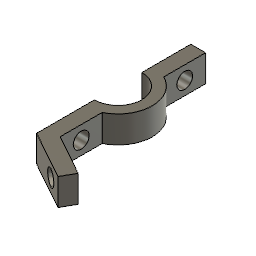
Trumpet+Clamp+1+Secondary (Autodesk Fusion 360 design; units mm, degrees)
Autodesk Fusion 360 part; units mm, degrees
sketch "Sketch1" plane through (0, 0, 0) normal (0, 1, 0) x (1, 0, 0)
  circle A0 centre (0, 0) radius 6.755
  circle A1 centre (0, 0) radius 9.755
  line L0 (0, 0) -> (-9.755, 0) construction
  line L1 (0, 0) -> (9.755, 0) construction
  line L2 (-4.25, -25.7687) -> (18.9274, -38.7154)
  line L3 (4.25, -20.7805) -> (23.0726, -31.2946)
  circle A2 centre (21, -35.005) radius 4.25
  line L4 (21, -35.005) -> (18.9274, -38.7154) construction
  line L5 (21, -35.005) -> (23.0726, -31.2946) construction
  circle A3 centre (21, -35.005) radius 2.25
  line L6 (-4.25, -25.7687) -> (-4.25, -8.7805)
  line L7 (4.25, -20.7805) -> (4.25, -8.7805)
  line L8 (0, 0) -> (0, -20.7805) construction
  line L9 (4.25, -20.7805) -> (-4.25, -20.7805) construction
  line L10 (-4.25, 8.7805) -> (-4.25, 20.7805)
  line L11 (-4.25, 20.7805) -> (4.25, 20.7805)
  line L12 (4.25, 20.7805) -> (4.25, 8.7805)
  line L13 (-4.25, -8.7805) -> (-4.25, 8.7805) construction
  line L14 (4.25, 8.7805) -> (4.25, -8.7805) construction
  line L15 (21, -35.005) -> (21, -39.255) construction
  point P0 (0, -9.755)
  point P1 (21, -39.255)
  dimension "d1" = 13.51
  dimension "d3" = 4.5
  dimension "d4" = 8.5
  dimension "d5" = 21
  dimension "d19" = 8.5
  dimension "d22" = 19.51
  dimension "d31" = 12
  dimension "d32" = 12
  dimension "d35" = 29.5
  constraint coincident A0.centre A1.centre
  constraint concentric A0 A1
  constraint coincident A1 L0.end
  constraint horizontal L0
  constraint coincident A1 L1.end
  constraint parallel L0 L1
  constraint coincident A2.centre L4.start
  constraint coincident A2 L2.end
  constraint coincident A2 L3.end
  constraint parallel L4 L5
  constraint coincident L2.end L4.end
  constraint coincident L3.end L5.end
  constraint coincident A1 L6.end
  constraint coincident A1 L7.end
  constraint parallel L2 L3
  constraint vertical L6
  constraint vertical L7
  constraint vertical L8
  constraint tangent L3 A2
  constraint coincident L6 L9.end
  constraint perpendicular L6 L9
  constraint midpoint L8.end L9
  constraint coincident A1 L10.start
  constraint vertical L10
  constraint perpendicular L10 L11
  constraint coincident A1 L12.end
  constraint perpendicular L11 L12
  constraint vertical L13
  constraint vertical L14
  constraint coincident L8 P0
  constraint coincident A1 P0
  constraint coincident A2 P1
  constraint vertical L15
  constraint coincident P1 L15.end
  measures "d1" diameter of A0
  measures "d3" diameter of A3
  measures "d4" diameter of A2
  measures "d5" horizontal distance of A0.centre A2.centre
  measures "d19" distance of L6 L7
  measures "d22" diameter of A1
  measures "d31" distance of L11.end L12.end
  measures "d32" distance of L3.start L7.end
  measures "d35" vertical distance of P0 P1
extrude "Extrude1" add sketch "Sketch1" along normal blind 7.7
sketch "Sketch2" plane through (-7.8365, 0, 14.0291) normal (0.487666, 0, -0.87303) x (-0.87303, 0, -0.487666)
  line L0 (-35.4044, 0) -> (-13.8443, 0)
  line L1 (-13.8443, 0) -> (-13.8443, 7.7)
  line L2 (-13.8443, 7.7) -> (-35.4044, 7.7)
  line L3 (-35.4044, 7.7) -> (-35.4044, 0)
  line L4 (-13.8443, 3.85) -> (-35.4044, 3.85) construction
  circle A0 centre (-21.8443, 3.85) radius 2.25
  dimension "d33" = 8
  dimension "d34" = 4.5
  constraint midpoint L1 L4.start
  constraint midpoint L3 L4.end
  constraint coincident L4 A0.centre
  measures "d33" distance of L1 A0.centre
  measures "d34" diameter of A0
extrude "Extrude2" cut sketch "Sketch2" against normal up to surface (8.5 mm away) contours A0
sketch "Sketch3" plane through (4.25, 0, 0) normal (1, 0, 0) x (0, 0, -1)
  line L0 (-20.7805, 0) -> (-8.7805, 0)
  line L1 (-8.7805, 0) -> (-8.7805, 7.7)
  line L2 (-8.7805, 7.7) -> (-20.7805, 7.7)
  line L3 (-20.7805, 7.7) -> (-20.7805, 0)
  line L4 (-8.7805, 3.85) -> (-20.7805, 3.85) construction
  circle A0 centre (-14.7805, 3.85) radius 2.25
  line L5 (8.7805, 0) -> (20.7805, 0) construction
  line L6 (20.7805, 0) -> (20.7805, 7.7) construction
  line L7 (20.7805, 7.7) -> (8.7805, 7.7) construction
  line L8 (8.7805, 7.7) -> (8.7805, 0) construction
  line L9 (8.7805, 3.85) -> (20.7805, 3.85) construction
  circle A1 centre (14.7805, 3.85) radius 2.25
  dimension "d16" = 4.5
  constraint midpoint L1 L4.start
  constraint midpoint L3 L4.end
  constraint midpoint L4 A0.centre
  constraint midpoint L8 L9.start
  constraint midpoint L6 L9.end
  constraint midpoint L9 A1.centre
  constraint equal A0 A1
  measures "d16" diameter of A0
extrude "Extrude3" cut sketch "Sketch3" against normal up to surface (8.5 mm away) contours A0 | A1
sketch "Sketch4" plane through (0, 0, 0) normal (1, 0, 0) x (0, 0, -1)
  circle A0 centre (-14.7805, 3.85) radius 2.25 construction
  line L0 (-20.7805, 0) -> (-8.7805, 0) construction
  line L1 (-8.7805, 0) -> (-8.7805, 7.7) construction
  line L2 (-8.7805, 7.7) -> (-20.7805, 7.7) construction
  line L3 (-20.7805, 7.7) -> (-20.7805, 0) construction
  line L4 (8.7805, 0) -> (-8.7805, 0) construction
  line L5 (-8.7805, 0) -> (-8.7805, 7.7) construction
  line L6 (8.7805, 7.7) -> (-8.7805, 7.7) construction
  line L7 (-8.7805, 7.7) -> (-8.7805, 0) construction
  circle A1 centre (-14.7805, 3.85) radius 2.25 construction
  line L8 (-8.7805, 0) -> (-25.7687, 0) construction
  line L9 (-25.7687, 0) -> (-25.7687, 7.7) construction
  line L10 (-25.7687, 7.7) -> (-8.7805, 7.7) construction
  line L11 (-8.7805, 7.7) -> (-8.7805, 0) construction
  line L12 (8.7805, 0) -> (-23.2746, 0)
  line L13 (-23.2746, 0) -> (-23.2746, 7.7)
  line L14 (-23.2746, 7.7) -> (8.7805, 7.7)
  line L15 (8.7805, 7.7) -> (8.7805, 0)
  line L16 (-25.7687, 7.7) -> (-20.7805, 7.7) construction
  line L17 (8.7805, 7.7) -> (8.7805, 0)
  line L18 (8.7805, 0) -> (-8.7805, 0)
  line L19 (8.7805, 0) -> (8.7805, 7.7)
  line L20 (8.7805, 7.7) -> (-8.7805, 7.7)
  circle A2 centre (14.7805, 3.85) radius 2.25
  line L21 (8.7805, 0) -> (20.7805, 0)
  line L22 (20.7805, 0) -> (20.7805, 7.7)
  line L23 (20.7805, 7.7) -> (8.7805, 7.7)
  line L24 (8.7805, 7.7) -> (8.7805, 0)
  constraint horizontal L12
  constraint vertical L13
  constraint horizontal L14
  constraint vertical L15
  constraint coincident L10 L13.end
  constraint coincident L4.start L12.start
  constraint coincident L9.end L10.start
  constraint coincident L2.end L3.start
  constraint midpoint L13.end L16
extrude "Extrude4" cut sketch "Sketch4" against normal blind 9.755
ref_plane "WorkPlane1" through (9.4113, 3.85, 28.5317) normal (-0.487666, 0, 0.87303) x (0.87303, 0, 0.487666)
sketch "Sketch5" plane through (-9.9091, 0, 17.7395) normal (-0.487666, 0, 0.87303) x (0.87303, 0, 0.487666)
  line L0 (7.6399, 0) -> (7.6399, 7.7)
  line L1 (7.6399, 7.7) -> (11.3502, 7.7)
  line L2 (11.3502, 7.7) -> (11.3502, 0)
  line L3 (11.3502, 0) -> (7.6399, 0)
  circle A0 centre (21.8443, 3.85) radius 2.25
  line L4 (35.4044, 0) -> (13.8443, 0)
  line L5 (13.8443, 0) -> (13.8443, 7.7)
  line L6 (13.8443, 7.7) -> (35.4044, 7.7)
  line L7 (35.4044, 7.7) -> (35.4044, 0)
  line L8 (7.6399, 7.7) -> (27.1402, 7.7)
  line L9 (27.1402, 7.7) -> (27.1402, 0)
  line L10 (27.1402, 0) -> (7.6399, 0)
  line L11 (7.6399, 0) -> (7.6399, 7.7)
  line L12 (21.8443, 3.85) -> (21.8443, 7.7) construction
  line L13 (21.8443, 7.7) -> (35.4044, 7.7) construction
  point P0 (27.1402, 8)
  dimension "d37" = 15.79
  constraint horizontal L8
  constraint vertical L9
  constraint horizontal L10
  constraint vertical L11
  constraint coincident L4 L9.end
  constraint coincident L0.end L1.start
  constraint coincident A0.centre L12.start
  constraint coincident L6 L12.end
  constraint vertical L12
  constraint coincident L6.end L7.start
  constraint coincident L9 P0
  measures "d37" distance of L2 L9
extrude "Extrude5" cut sketch "Sketch5" along normal up to surface (4.25 mm away) contours L0 L1 L2 L3 L8 L10 L11 | L2 L5 L8 L10 | L4 L5 L6 L8 L9 L10
sketch "Sketch6" plane through (-11.9817, 0, 21.4499) normal (-0.487666, 0, 0.87303) x (0.87303, 0, 0.487666)
  line L0 (27.1402, 7.7) -> (27.1402, 0)
  line L1 (27.1402, 0) -> (35.4044, 0)
  line L2 (35.4044, 0) -> (35.4044, 7.7)
  line L3 (35.4044, 7.7) -> (27.1402, 7.7)
  line L4 (39.6544, 0) -> (35.4044, 0)
  line L5 (35.4044, 0) -> (35.4044, 7.7)
  line L6 (39.6544, 7.7) -> (35.4044, 7.7)
  line L7 (27.1402, 7.7) -> (39.6544, 7.7)
  line L8 (39.6544, 7.7) -> (39.6544, 0)
  line L9 (39.6544, 0) -> (27.1402, 0)
  line L10 (27.1402, 0) -> (27.1402, 7.7)
  line L11 (35.4044, 7.7) -> (35.4044, 0)
  constraint horizontal L7
  constraint vertical L8
  constraint horizontal L9
  constraint vertical L10
  constraint coincident L4.start L8.end
  constraint coincident L0.start L3.end
extrude "Extrude6" cut sketch "Sketch6" against normal up to surface (8.5 mm away)
equation "d19 = d4"
equation "d20 = ( -d22 / 2 mm ) * 1 mm"
equation "d22 = d1 + 6 mm"
equation "d31 = d32"
